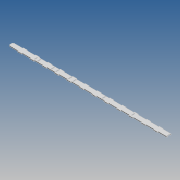
# Autodesk Inventor part: CaissonLongueur
Saved by Autodesk Inventor 2019 (Build 230136000, 136)
## iProperties
Created: 2019-08-26
Part Number: CaissonLongueur
Material: PVC-U
Document SubType Name: Modeling
Designer: jeremias.salamin
Density: 1.4 g/cm^3
Appearance: Lisse - Blanc
Description: CaissonLongueur
Author: jeremias.salamin
Autodesk Inventor part; units mm, degrees
ref_plane "YZ Plane" through (0, 0, 0) normal (1, 0, 0) x (0, 1, 0)
ref_plane "XZ Plane" through (0, 0, 0) normal (0, 1, 0) x (-1, 0, 0)
ref_plane "XY Plane" through (0, 0, 0) normal (0, 0, 1) x (1, 0, 0)
sketch "Sketch1" plane through (0, 0, 0) normal (0, 0, 1) x (1, 0, 0)
  line L0 (0, 6.16) -> (0, -6.16) construction
  line L1 (-222.88, 0) -> (222.88, 0) construction
  line L2 (159.2, -4.4) -> (-159.2, -4.4)
  line L3 (-159.2, -4.4) -> (-159.2, 4.4)
  line L4 (-159.2, 4.4) -> (159.2, 4.4)
  line L5 (159.2, 4.4) -> (159.2, -4.4)
  line L6 (159.2, -4.4) -> (-159.2, 4.4) construction
  line L7 (-159.2, -4.4) -> (159.2, 4.4) construction
  point P0 (0, 0)
  dimension "d0" = 8.8
  dimension "d1" = 318.4
  constraints: 12 end point, 2 midpoint, 2 parallel, 1 horizontal, 1 perpendicular
  measures "d0" distance of L2.end L3.end
  measures "d1" distance of L3.end L4.end
extrude "Extrusion1" add sketch "Sketch1" along normal mid plane 1.6
sketch "Esquisse3" plane through (0, 0, -0.8) normal (0, 0, -1) x (-1, 0, 0)
  line L0 (-85.6, -3) -> (-87.2, -3)
  line L1 (-87.2, -3) -> (-87.2, 3)
  line L2 (-87.2, 3) -> (-85.6, 3)
  line L3 (-85.6, 3) -> (-85.6, -3)
  line L4 (-157.6, -3) -> (-159.2, -3)
  line L5 (-159.2, -3) -> (-159.2, 3)
  line L6 (-159.2, 3) -> (-157.6, 3)
  line L7 (-157.6, 3) -> (-157.6, -3)
  line L8 (-26.3, -3) -> (-27.9, -3)
  line L9 (-27.9, -3) -> (-27.9, 3)
  line L10 (-27.9, 3) -> (-26.3, 3)
  line L11 (-26.3, 3) -> (-26.3, -3)
  line L12 (109.2, 3) -> (110.8, 3)
  line L13 (110.8, 3) -> (110.8, -3)
  line L14 (110.8, -3) -> (109.2, -3)
  line L15 (109.2, -3) -> (109.2, 3)
  line L16 (75, 3) -> (76.6, 3)
  line L17 (76.6, 3) -> (76.6, -3)
  line L18 (76.6, -3) -> (75, -3)
  line L19 (75, -3) -> (75, 3)
  line L20 (33, -3) -> (31.4, -3)
  line L21 (31.4, -3) -> (31.4, 3)
  line L22 (31.4, 3) -> (33, 3)
  line L23 (33, 3) -> (33, -3)
  point P0 (0, 0)
  constraints: 48 end point, 12 horizontal, 12 vertical, 24 other
extrude "Extrusion4" cut sketch "Esquisse3" against normal blind 1.6
sketch "Esquisse4" plane through (0, 0, 0.8) normal (0, 0, 1) x (1, 0, 0)
  line L0 (-102.6, -3) -> (-104.2, -3)
  line L1 (-104.2, -3) -> (-104.2, 3)
  line L2 (-104.2, 3) -> (-102.6, 3)
  line L3 (-102.6, 3) -> (-102.6, -3)
  line L4 (-66, -3) -> (-67.6, -3)
  line L5 (-67.6, -3) -> (-67.6, 3)
  line L6 (-67.6, 3) -> (-66, 3)
  line L7 (-66, 3) -> (-66, -3)
  line L8 (-42.4, 3) -> (-40.8, 3)
  line L9 (-40.8, 3) -> (-40.8, -3)
  line L10 (-40.8, -3) -> (-42.4, -3)
  line L11 (-42.4, -3) -> (-42.4, 3)
  point P0 (0, 0)
  constraints: 24 end point, 6 horizontal, 6 vertical, 12 other
extrude "Extrusion5" cut sketch "Esquisse4" against normal blind 1.6
sketch "Esquisse5" plane through (0, 0, 0.8) normal (0, 0, 1) x (1, 0, 0)
  line L0 (-66, 3) -> (-66, -3) construction
  line L1 (-66, -3) -> (-67.6, -3) construction
  line L2 (-67.6, -3) -> (-67.6, 3) construction
  line L3 (-67.6, 3) -> (-66, 3) construction
  line L4 (-102.6, 3) -> (-102.6, -3) construction
  line L5 (-102.6, -3) -> (-104.2, -3) construction
  line L6 (-104.2, -3) -> (-104.2, 3) construction
  line L7 (-104.2, 3) -> (-102.6, 3) construction
  line L8 (-42.4, -3) -> (-42.4, 3) construction
  line L9 (-42.4, 3) -> (-40.8, 3) construction
  line L10 (-40.8, 3) -> (-40.8, -3) construction
  line L11 (-40.8, -3) -> (-42.4, -3) construction
  line L12 (157.6, 3) -> (159.2, 3) construction
  line L13 (159.2, 3) -> (159.2, 4.4) construction
  line L14 (159.2, 4.4) -> (-159.2, 4.4) construction
  line L15 (-159.2, 4.4) -> (-159.2, -4.4) construction
  line L16 (-159.2, -4.4) -> (159.2, -4.4) construction
  line L17 (159.2, -4.4) -> (159.2, -3) construction
  line L18 (159.2, -3) -> (157.6, -3) construction
  line L19 (157.6, -3) -> (157.6, 3) construction
  line L20 (-75, 3) -> (-75, -3) construction
  line L21 (-75, -3) -> (-76.6, -3) construction
  line L22 (-76.6, -3) -> (-76.6, 3) construction
  line L23 (-76.6, 3) -> (-75, 3) construction
  line L24 (26.3, -3) -> (26.3, 3) construction
  line L25 (26.3, 3) -> (27.9, 3) construction
  line L26 (27.9, 3) -> (27.9, -3) construction
  line L27 (27.9, -3) -> (26.3, -3) construction
  line L28 (85.6, -3) -> (85.6, 3) construction
  line L29 (85.6, 3) -> (87.2, 3) construction
  line L30 (87.2, 3) -> (87.2, -3) construction
  line L31 (87.2, -3) -> (85.6, -3) construction
  line L32 (-109.2, 3) -> (-109.2, -3) construction
  line L33 (-109.2, -3) -> (-110.8, -3) construction
  line L34 (-110.8, -3) -> (-110.8, 3) construction
  line L35 (-110.8, 3) -> (-109.2, 3) construction
  line L36 (-33, -3) -> (-33, 3) construction
  line L37 (-33, 3) -> (-31.4, 3) construction
  line L38 (-31.4, 3) -> (-31.4, -3) construction
  line L39 (-31.4, -3) -> (-33, -3) construction
  line L40 (0, 6.16) -> (0, -6.16) construction
  line L41 (-222.88, 0) -> (222.88, 0) construction
  line L42 (-141.5, 4.4) -> (-133.5, 4.4)
  line L43 (-133.5, 4.4) -> (-133.5, 6)
  line L44 (-133.5, 6) -> (-141.5, 6)
  line L45 (-141.5, 6) -> (-141.5, 4.4)
  line L46 (-108.5, 4.4) -> (-108.5, 6)
  line L47 (-108.5, 6) -> (-116.5, 6)
  line L48 (-116.5, 6) -> (-116.5, 4.4)
  line L49 (-116.5, 4.4) -> (-108.5, 4.4)
  line L50 (-83.5, 4.4) -> (-83.5, 6)
  line L51 (-83.5, 6) -> (-91.5, 6)
  line L52 (-91.5, 6) -> (-91.5, 4.4)
  line L53 (-91.5, 4.4) -> (-83.5, 4.4)
  line L54 (-58.5, 4.4) -> (-58.5, 6)
  line L55 (-58.5, 6) -> (-66.5, 6)
  line L56 (-66.5, 6) -> (-66.5, 4.4)
  line L57 (-66.5, 4.4) -> (-58.5, 4.4)
  line L58 (-33.5, 4.4) -> (-33.5, 6)
  line L59 (-33.5, 6) -> (-41.5, 6)
  line L60 (-41.5, 6) -> (-41.5, 4.4)
  line L61 (-41.5, 4.4) -> (-33.5, 4.4)
  line L62 (-8.5, 4.4) -> (-8.5, 6)
  line L63 (-8.5, 6) -> (-16.5, 6)
  line L64 (-16.5, 6) -> (-16.5, 4.4)
  line L65 (-16.5, 4.4) -> (-8.5, 4.4)
  line L66 (16.5, 4.4) -> (16.5, 6)
  line L67 (16.5, 6) -> (8.5, 6)
  line L68 (8.5, 6) -> (8.5, 4.4)
  line L69 (8.5, 4.4) -> (16.5, 4.4)
  line L70 (41.5, 4.4) -> (41.5, 6)
  line L71 (41.5, 6) -> (33.5, 6)
  line L72 (33.5, 6) -> (33.5, 4.4)
  line L73 (33.5, 4.4) -> (41.5, 4.4)
  line L74 (66.5, 4.4) -> (66.5, 6)
  line L75 (66.5, 6) -> (58.5, 6)
  line L76 (58.5, 6) -> (58.5, 4.4)
  line L77 (58.5, 4.4) -> (66.5, 4.4)
  line L78 (91.5, 4.4) -> (91.5, 6)
  line L79 (91.5, 6) -> (83.5, 6)
  line L80 (83.5, 6) -> (83.5, 4.4)
  line L81 (83.5, 4.4) -> (91.5, 4.4)
  line L82 (116.5, 4.4) -> (116.5, 6)
  line L83 (116.5, 6) -> (108.5, 6)
  line L84 (108.5, 6) -> (108.5, 4.4)
  line L85 (108.5, 4.4) -> (116.5, 4.4)
  line L86 (141.5, 4.4) -> (141.5, 6)
  line L87 (141.5, 6) -> (133.5, 6)
  line L88 (133.5, 6) -> (133.5, 4.4)
  line L89 (133.5, 4.4) -> (141.5, 4.4)
  point P0 (0, 0)
  dimension "d21" = 8
  dimension "d22" = 1.6
  dimension "d25" = 25
  constraints: 96 end point, 2 horizontal, 2 parallel, 1 perpendicular, 1 point on line, 89 other
  measures "d21" distance of L44.end L43.end
  measures "d22" distance of L43.end L42.end
  measures "d25" distance of L42.end L46.start
extrude "Extrusion6" add sketch "Esquisse5" against normal blind 1.6
mirror "Symétrie2" about plane through (0, 0, 0) normal (0, 1, 0) of "Extrusion6"
sketch "Esquisse6" plane through (0, 0, 0.8) normal (0, 0, 1) x (1, 0, 0)
  line L0 (-66, -3) -> (-66, 3) construction
  line L1 (-66, 3) -> (-67.6, 3) construction
  line L2 (-67.6, 3) -> (-67.6, -3) construction
  line L3 (-67.6, -3) -> (-66, -3) construction
  line L4 (-102.6, -3) -> (-102.6, 3) construction
  line L5 (-102.6, 3) -> (-104.2, 3) construction
  line L6 (-104.2, 3) -> (-104.2, -3) construction
  line L7 (-104.2, -3) -> (-102.6, -3) construction
  line L8 (-42.4, 3) -> (-42.4, -3) construction
  line L9 (-42.4, -3) -> (-40.8, -3) construction
  line L10 (-40.8, -3) -> (-40.8, 3) construction
  line L11 (-40.8, 3) -> (-42.4, 3) construction
  line L12 (-75, -3) -> (-75, 3) construction
  line L13 (-75, 3) -> (-76.6, 3) construction
  line L14 (-76.6, 3) -> (-76.6, -3) construction
  line L15 (-76.6, -3) -> (-75, -3) construction
  line L16 (26.3, 3) -> (26.3, -3) construction
  line L17 (26.3, -3) -> (27.9, -3) construction
  line L18 (27.9, -3) -> (27.9, 3) construction
  line L19 (27.9, 3) -> (26.3, 3) construction
  line L20 (85.6, 3) -> (85.6, -3) construction
  line L21 (85.6, -3) -> (87.2, -3) construction
  line L22 (87.2, -3) -> (87.2, 3) construction
  line L23 (87.2, 3) -> (85.6, 3) construction
  line L24 (157.6, 3) -> (157.6, -3) construction
  line L25 (157.6, -3) -> (159.2, -3) construction
  line L26 (159.2, -3) -> (159.2, -4.4) construction
  line L27 (159.2, -4.4) -> (141.5, -4.4) construction
  line L28 (141.5, -4.4) -> (141.5, -6) construction
  line L29 (141.5, -6) -> (133.5, -6) construction
  line L30 (133.5, -6) -> (133.5, -4.4) construction
  line L31 (133.5, -4.4) -> (116.5, -4.4) construction
  line L32 (116.5, -4.4) -> (116.5, -6) construction
  line L33 (116.5, -6) -> (108.5, -6) construction
  line L34 (108.5, -6) -> (108.5, -4.4) construction
  line L35 (108.5, -4.4) -> (91.5, -4.4) construction
  line L36 (91.5, -4.4) -> (91.5, -6) construction
  line L37 (91.5, -6) -> (83.5, -6) construction
  line L38 (83.5, -6) -> (83.5, -4.4) construction
  line L39 (83.5, -4.4) -> (66.5, -4.4) construction
  line L40 (66.5, -4.4) -> (66.5, -6) construction
  line L41 (66.5, -6) -> (58.5, -6) construction
  line L42 (58.5, -6) -> (58.5, -4.4) construction
  line L43 (58.5, -4.4) -> (41.5, -4.4) construction
  line L44 (41.5, -4.4) -> (41.5, -6) construction
  line L45 (41.5, -6) -> (33.5, -6) construction
  line L46 (33.5, -6) -> (33.5, -4.4) construction
  line L47 (33.5, -4.4) -> (16.5, -4.4) construction
  line L48 (16.5, -4.4) -> (16.5, -6) construction
  line L49 (16.5, -6) -> (8.5, -6) construction
  line L50 (8.5, -6) -> (8.5, -4.4) construction
  line L51 (8.5, -4.4) -> (-8.5, -4.4) construction
  line L52 (-8.5, -4.4) -> (-8.5, -6) construction
  line L53 (-8.5, -6) -> (-16.5, -6) construction
  line L54 (-16.5, -6) -> (-16.5, -4.4) construction
  line L55 (-16.5, -4.4) -> (-33.5, -4.4) construction
  line L56 (-33.5, -4.4) -> (-33.5, -6) construction
  line L57 (-33.5, -6) -> (-41.5, -6) construction
  line L58 (-41.5, -6) -> (-41.5, -4.4) construction
  line L59 (-41.5, -4.4) -> (-58.5, -4.4) construction
  line L60 (-58.5, -4.4) -> (-58.5, -6) construction
  line L61 (-58.5, -6) -> (-66.5, -6) construction
  line L62 (-66.5, -6) -> (-66.5, -4.4) construction
  line L63 (-66.5, -4.4) -> (-83.5, -4.4) construction
  line L64 (-83.5, -4.4) -> (-83.5, -6) construction
  line L65 (-83.5, -6) -> (-91.5, -6) construction
  line L66 (-91.5, -6) -> (-91.5, -4.4) construction
  line L67 (-91.5, -4.4) -> (-108.5, -4.4) construction
  line L68 (-108.5, -4.4) -> (-108.5, -6) construction
  line L69 (-108.5, -6) -> (-116.5, -6) construction
  line L70 (-116.5, -6) -> (-116.5, -4.4) construction
  line L71 (-116.5, -4.4) -> (-133.5, -4.4) construction
  line L72 (-133.5, -4.4) -> (-133.5, -6) construction
  line L73 (-133.5, -6) -> (-141.5, -6) construction
  line L74 (-141.5, -6) -> (-141.5, -4.4) construction
  line L75 (-141.5, -4.4) -> (-159.2, -4.4) construction
  line L76 (-159.2, -4.4) -> (-159.2, 4.4) construction
  line L77 (-159.2, 4.4) -> (-141.5, 4.4) construction
  line L78 (-141.5, 4.4) -> (-141.5, 6) construction
  line L79 (-141.5, 6) -> (-133.5, 6) construction
  line L80 (-133.5, 6) -> (-133.5, 4.4) construction
  line L81 (-133.5, 4.4) -> (-116.5, 4.4) construction
  line L82 (-116.5, 4.4) -> (-116.5, 6) construction
  line L83 (-116.5, 6) -> (-108.5, 6) construction
  line L84 (-108.5, 6) -> (-108.5, 4.4) construction
  line L85 (-108.5, 4.4) -> (-91.5, 4.4) construction
  line L86 (-91.5, 4.4) -> (-91.5, 6) construction
  line L87 (-91.5, 6) -> (-83.5, 6) construction
  line L88 (-83.5, 6) -> (-83.5, 4.4) construction
  line L89 (-83.5, 4.4) -> (-66.5, 4.4) construction
  line L90 (-66.5, 4.4) -> (-66.5, 6) construction
  line L91 (-66.5, 6) -> (-58.5, 6) construction
  line L92 (-58.5, 6) -> (-58.5, 4.4) construction
  line L93 (-58.5, 4.4) -> (-41.5, 4.4) construction
  line L94 (-41.5, 4.4) -> (-41.5, 6) construction
  line L95 (-41.5, 6) -> (-33.5, 6) construction
  line L96 (-33.5, 6) -> (-33.5, 4.4) construction
  line L97 (-33.5, 4.4) -> (-16.5, 4.4) construction
  line L98 (-16.5, 4.4) -> (-16.5, 6) construction
  line L99 (-16.5, 6) -> (-8.5, 6) construction
  line L100 (-8.5, 6) -> (-8.5, 4.4) construction
  line L101 (-8.5, 4.4) -> (8.5, 4.4) construction
  line L102 (8.5, 4.4) -> (8.5, 6) construction
  line L103 (8.5, 6) -> (16.5, 6) construction
  line L104 (16.5, 6) -> (16.5, 4.4) construction
  line L105 (16.5, 4.4) -> (33.5, 4.4) construction
  line L106 (33.5, 4.4) -> (33.5, 6) construction
  line L107 (33.5, 6) -> (41.5, 6) construction
  line L108 (41.5, 6) -> (41.5, 4.4) construction
  line L109 (41.5, 4.4) -> (58.5, 4.4) construction
  line L110 (58.5, 4.4) -> (58.5, 6) construction
  line L111 (58.5, 6) -> (66.5, 6) construction
  line L112 (66.5, 6) -> (66.5, 4.4) construction
  line L113 (66.5, 4.4) -> (83.5, 4.4) construction
  line L114 (83.5, 4.4) -> (83.5, 6) construction
  line L115 (83.5, 6) -> (91.5, 6) construction
  line L116 (91.5, 6) -> (91.5, 4.4) construction
  line L117 (91.5, 4.4) -> (108.5, 4.4) construction
  line L118 (108.5, 4.4) -> (108.5, 6) construction
  line L119 (108.5, 6) -> (116.5, 6) construction
  line L120 (116.5, 6) -> (116.5, 4.4) construction
  line L121 (116.5, 4.4) -> (133.5, 4.4) construction
  line L122 (133.5, 4.4) -> (133.5, 6) construction
  line L123 (133.5, 6) -> (141.5, 6) construction
  line L124 (141.5, 6) -> (141.5, 4.4) construction
  line L125 (141.5, 4.4) -> (159.2, 4.4) construction
  line L126 (159.2, 4.4) -> (159.2, 3) construction
  line L127 (159.2, 3) -> (157.6, 3) construction
  line L128 (-109.2, -3) -> (-109.2, 3) construction
  line L129 (-109.2, 3) -> (-110.8, 3) construction
  line L130 (-110.8, 3) -> (-110.8, -3) construction
  line L131 (-110.8, -3) -> (-109.2, -3) construction
  line L132 (-33, 3) -> (-33, -3) construction
  line L133 (-33, -3) -> (-31.4, -3) construction
  line L134 (-31.4, -3) -> (-31.4, 3) construction
  line L135 (-31.4, 3) -> (-33, 3) construction
  line L136 (-66, 3) -> (-66, -3) construction
  line L137 (-66, -3) -> (-67.6, -3) construction
  line L138 (-67.6, -3) -> (-67.6, 3) construction
  line L139 (-67.6, 3) -> (-66, 3) construction
  line L140 (-102.6, 3) -> (-102.6, -3) construction
  line L141 (-102.6, -3) -> (-104.2, -3) construction
  line L142 (-104.2, -3) -> (-104.2, 3) construction
  line L143 (-104.2, 3) -> (-102.6, 3) construction
  line L144 (-42.4, -3) -> (-42.4, 3) construction
  line L145 (-42.4, 3) -> (-40.8, 3) construction
  line L146 (-40.8, 3) -> (-40.8, -3) construction
  line L147 (-40.8, -3) -> (-42.4, -3) construction
  line L148 (157.6, 3) -> (159.2, 3) construction
  line L149 (159.2, 3) -> (159.2, 4.4) construction
  line L150 (159.2, 4.4) -> (141.5, 4.4) construction
  line L151 (141.5, 6) -> (141.5, 4.4) construction
  line L152 (133.5, 6) -> (141.5, 6) construction
  line L153 (133.5, 4.4) -> (133.5, 6) construction
  line L154 (133.5, 4.4) -> (116.5, 4.4) construction
  line L155 (116.5, 6) -> (116.5, 4.4) construction
  line L156 (108.5, 6) -> (116.5, 6) construction
  line L157 (108.5, 4.4) -> (108.5, 6) construction
  line L158 (108.5, 4.4) -> (91.5, 4.4) construction
  line L159 (91.5, 6) -> (91.5, 4.4) construction
  line L160 (83.5, 6) -> (91.5, 6) construction
  line L161 (83.5, 4.4) -> (83.5, 6) construction
  line L162 (83.5, 4.4) -> (66.5, 4.4) construction
  line L163 (66.5, 6) -> (66.5, 4.4) construction
  line L164 (58.5, 6) -> (66.5, 6) construction
  line L165 (58.5, 4.4) -> (58.5, 6) construction
  line L166 (58.5, 4.4) -> (41.5, 4.4) construction
  line L167 (41.5, 6) -> (41.5, 4.4) construction
  line L168 (33.5, 6) -> (41.5, 6) construction
  line L169 (33.5, 4.4) -> (33.5, 6) construction
  line L170 (33.5, 4.4) -> (16.5, 4.4) construction
  line L171 (16.5, 6) -> (16.5, 4.4) construction
  line L172 (8.5, 6) -> (16.5, 6) construction
  line L173 (8.5, 4.4) -> (8.5, 6) construction
  line L174 (8.5, 4.4) -> (-8.5, 4.4) construction
  line L175 (-8.5, 6) -> (-8.5, 4.4) construction
  line L176 (-16.5, 6) -> (-8.5, 6) construction
  line L177 (-16.5, 4.4) -> (-16.5, 6) construction
  line L178 (-16.5, 4.4) -> (-33.5, 4.4) construction
  line L179 (-33.5, 6) -> (-33.5, 4.4) construction
  line L180 (-41.5, 6) -> (-33.5, 6) construction
  line L181 (-41.5, 4.4) -> (-41.5, 6) construction
  line L182 (-41.5, 4.4) -> (-58.5, 4.4) construction
  line L183 (-58.5, 6) -> (-58.5, 4.4) construction
  line L184 (-66.5, 6) -> (-58.5, 6) construction
  line L185 (-66.5, 4.4) -> (-66.5, 6) construction
  line L186 (-66.5, 4.4) -> (-83.5, 4.4) construction
  line L187 (-83.5, 6) -> (-83.5, 4.4) construction
  line L188 (-91.5, 6) -> (-83.5, 6) construction
  line L189 (-91.5, 4.4) -> (-91.5, 6) construction
  line L190 (-91.5, 4.4) -> (-108.5, 4.4) construction
  line L191 (-108.5, 6) -> (-108.5, 4.4) construction
  line L192 (-116.5, 6) -> (-108.5, 6) construction
  line L193 (-116.5, 4.4) -> (-116.5, 6) construction
  line L194 (-116.5, 4.4) -> (-133.5, 4.4) construction
  line L195 (-133.5, 4.4) -> (-133.5, 6) construction
  line L196 (-133.5, 6) -> (-141.5, 6) construction
  line L197 (-141.5, 6) -> (-141.5, 4.4) construction
  line L198 (-141.5, 4.4) -> (-159.2, 4.4) construction
  line L199 (-159.2, 4.4) -> (-159.2, -4.4) construction
  line L200 (-159.2, -4.4) -> (-141.5, -4.4) construction
  line L201 (-141.5, -6) -> (-141.5, -4.4) construction
  line L202 (-133.5, -6) -> (-141.5, -6) construction
  line L203 (-133.5, -4.4) -> (-133.5, -6) construction
  line L204 (-133.5, -4.4) -> (-116.5, -4.4) construction
  line L205 (-116.5, -4.4) -> (-116.5, -6) construction
  line L206 (-116.5, -6) -> (-108.5, -6) construction
  line L207 (-108.5, -6) -> (-108.5, -4.4) construction
  line L208 (-108.5, -4.4) -> (-91.5, -4.4) construction
  line L209 (-91.5, -4.4) -> (-91.5, -6) construction
  line L210 (-91.5, -6) -> (-83.5, -6) construction
  line L211 (-83.5, -6) -> (-83.5, -4.4) construction
  line L212 (-83.5, -4.4) -> (-66.5, -4.4) construction
  line L213 (-66.5, -4.4) -> (-66.5, -6) construction
  line L214 (-66.5, -6) -> (-58.5, -6) construction
  line L215 (-58.5, -6) -> (-58.5, -4.4) construction
  line L216 (-58.5, -4.4) -> (-41.5, -4.4) construction
  line L217 (-41.5, -4.4) -> (-41.5, -6) construction
  line L218 (-41.5, -6) -> (-33.5, -6) construction
  line L219 (-33.5, -6) -> (-33.5, -4.4) construction
  line L220 (-33.5, -4.4) -> (-16.5, -4.4) construction
  line L221 (-16.5, -4.4) -> (-16.5, -6) construction
  line L222 (-16.5, -6) -> (-8.5, -6) construction
  line L223 (-8.5, -6) -> (-8.5, -4.4) construction
  line L224 (-8.5, -4.4) -> (8.5, -4.4) construction
  line L225 (8.5, -4.4) -> (8.5, -6) construction
  line L226 (8.5, -6) -> (16.5, -6) construction
  line L227 (16.5, -6) -> (16.5, -4.4) construction
  line L228 (16.5, -4.4) -> (33.5, -4.4) construction
  line L229 (33.5, -4.4) -> (33.5, -6) construction
  line L230 (33.5, -6) -> (41.5, -6) construction
  line L231 (41.5, -6) -> (41.5, -4.4) construction
  line L232 (41.5, -4.4) -> (58.5, -4.4) construction
  line L233 (58.5, -4.4) -> (58.5, -6) construction
  line L234 (58.5, -6) -> (66.5, -6) construction
  line L235 (66.5, -6) -> (66.5, -4.4) construction
  line L236 (66.5, -4.4) -> (83.5, -4.4) construction
  line L237 (83.5, -4.4) -> (83.5, -6) construction
  line L238 (83.5, -6) -> (91.5, -6) construction
  line L239 (91.5, -6) -> (91.5, -4.4) construction
  line L240 (91.5, -4.4) -> (108.5, -4.4) construction
  line L241 (108.5, -4.4) -> (108.5, -6) construction
  line L242 (108.5, -6) -> (116.5, -6) construction
  line L243 (116.5, -6) -> (116.5, -4.4) construction
  line L244 (116.5, -4.4) -> (133.5, -4.4) construction
  line L245 (133.5, -4.4) -> (133.5, -6) construction
  line L246 (133.5, -6) -> (141.5, -6) construction
  line L247 (141.5, -6) -> (141.5, -4.4) construction
  line L248 (141.5, -4.4) -> (159.2, -4.4) construction
  line L249 (159.2, -4.4) -> (159.2, -3) construction
  line L250 (159.2, -3) -> (157.6, -3) construction
  line L251 (157.6, -3) -> (157.6, 3) construction
  line L252 (-75, 3) -> (-75, -3) construction
  line L253 (-75, -3) -> (-76.6, -3) construction
  line L254 (-76.6, -3) -> (-76.6, 3) construction
  line L255 (-76.6, 3) -> (-75, 3) construction
  line L256 (26.3, -3) -> (26.3, 3) construction
  line L257 (26.3, 3) -> (27.9, 3) construction
  line L258 (27.9, 3) -> (27.9, -3) construction
  line L259 (27.9, -3) -> (26.3, -3) construction
  line L260 (85.6, -3) -> (85.6, 3) construction
  line L261 (85.6, 3) -> (87.2, 3) construction
  line L262 (87.2, 3) -> (87.2, -3) construction
  line L263 (87.2, -3) -> (85.6, -3) construction
  line L264 (-109.2, 3) -> (-109.2, -3) construction
  line L265 (-109.2, -3) -> (-110.8, -3) construction
  line L266 (-110.8, -3) -> (-110.8, 3) construction
  line L267 (-110.8, 3) -> (-109.2, 3) construction
  line L268 (-33, -3) -> (-33, 3) construction
  line L269 (-33, 3) -> (-31.4, 3) construction
  line L270 (-31.4, 3) -> (-31.4, -3) construction
  line L271 (-31.4, -3) -> (-33, -3) construction
  line L272 (0, 8.4) -> (0, -8.4) construction
  line L273 (-222.88, 0) -> (222.88, 0) construction
  line L274 (-159.2, 3) -> (-160.8, 3)
  line L275 (-160.8, 3) -> (-160.8, -3)
  line L276 (-160.8, -3) -> (-159.2, -3)
  line L277 (-159.2, -3) -> (-159.2, 3)
  point P0 (0, 0)
  dimension "d32" = 1.6
  dimension "d33" = 6
  constraints: 8 end point, 2 parallel, 1 horizontal, 1 perpendicular, 1 point on line, 1 other
  measures "d32" distance of L276.end L275.end
  measures "d33" distance of L275.end L274.end
extrude "Extrusion7" add sketch "Esquisse6" against normal blind 1.6
